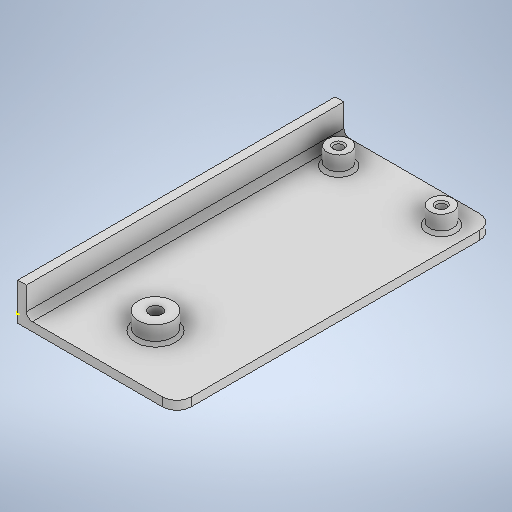
# Autodesk Inventor part: long_protoboard_backplate
Saved by Autodesk Inventor 2025.2 (Build 292293000, 293)
## iProperties
Created: 2025-03-28
Part Number: long_protoboard_backplate
Material: Generic
Document SubType Name: Modeling
Designer: osmon
Density: 1 g/cm^3
Appearance: Default
Author: osmon
Autodesk Inventor part; units mm, degrees
ref_plane "YZ Plane" through (0, 0, 0) normal (1, 0, 0) x (0, 1, 0)
ref_plane "XZ Plane" through (0, 0, 0) normal (0, 1, 0) x (-1, 0, 0)
ref_plane "XY Plane" through (0, 0, 0) normal (0, 0, 1) x (1, 0, 0)
sketch "Sketch1" plane through (0, 0, 0) normal (0, 1, 0) x (-1, 0, 0)
  line L0 (0, 0) -> (-55.1, 0)
  line L1 (-55.1, 0) -> (-55.1, -110)
  line L2 (-55.1, -110) -> (0, -110)
  line L3 (0, -110) -> (0, 0)
  dimension "d0" = 110
  dimension "d28" = 55.1
  constraints: 8 end point, 2 parallel, 1 horizontal, 1 perpendicular
  measures "d0" distance of L1.end L0.end
  measures "d28" distance of L1.end L2.end
extrude "Extrusion1" add sketch "Sketch1" along normal blind 3
sketch "Sketch2" plane through (0, 3, 0) normal (0, 1, 0) x (1, 0, 0)
  line L0 (55.1, 0) -> (55.1, 110) projected
  line L1 (55.1, 110) -> (0, 110) projected
  line L2 (0, 110) -> (0, 0) projected
  line L3 (0, 0) -> (55.1, 0) projected
  circle A0 centre (11.25, 99.95) radius 4
  circle A1 centre (46.85, 99.95) radius 4
  circle A2 centre (29.05, 18.6623) radius 6
  point P0 (27.55, 110)
  dimension "d3" = 8
  dimension "d4" = 10.05
  dimension "d6" = 8
  dimension "d7" = 10.05
  dimension "d8" = 8.25
  dimension "d29" = 12
  dimension "d30" = 91.35
  dimension "d39" = 26.05
  dimension "d40" = 35.6
  constraints: 3 centre point, 1 midpoint
  measures "d3" diameter of A0
  measures "d4" distance from line of L1 A0.centre
  measures "d6" diameter of A1
  measures "d7" distance from line of L1 A1.centre
  measures "d8" distance from line of L0 A1.centre
  measures "d29" diameter of A2
  measures "d30" distance of point (27.55, 110) A2.centre
  measures "d39" distance from line of L0 A2.centre
  measures "d40" distance of A1.centre A0.centre
extrude "Extrusion2" cut sketch "Sketch2" against normal blind 0.5 contours A0 | A1 | A2
sketch "Sketch3" plane through (11.25, 2.5, -99.95) normal (0, 1, 0) x (1, 0, 0)
  circle A0 centre (0, 0) radius 4 projected
  circle A1 centre (0, 0) radius 4
  circle A2 centre (35.6, 0) radius 4 projected
  circle A3 centre (35.6, 0) radius 4
  circle A4 centre (17.8, -81.2877) radius 6 projected
  circle A5 centre (17.8, -81.2877) radius 6
  point P0 (-11.25, -99.95)
  dimension "d32" = 12
  constraints: 3 centre point, 3 coincident, 2 concentric
  measures "d32" diameter of A5
extrude "Extrusion3" add sketch "Sketch3" along normal blind 6.5
sketch "Sketch4" plane through (11.25, 9, -99.95) normal (0, 1, 0) x (1, 0, 0)
  circle A0 centre (0, 0) radius 4 projected
  circle A1 centre (0, 0) radius 1.5
  circle A2 centre (35.6, 0) radius 4 projected
  circle A3 centre (35.6, 0) radius 1.5
  point P0 (-11.25, -99.95)
  dimension "d13" = 3
  dimension "d14" = 3
  constraints: 2 centre point, 2 coincident
  measures "d13" diameter of A1
  measures "d14" diameter of A3
extrude "Extrusion4" cut sketch "Sketch4" against normal blind 3.7 contours A1 | A3
chamfer "Chamfer1" distance 1 angle 45 3 edges at (7.25, 3, -99.95) (42.85, 3, -99.95) (23.05, 3, -18.6623)
chamfer "Chamfer2" distance 0.5 angle 45 2 edges at (9.75, 9, -99.95) (45.35, 9, -99.95)
sketch "Sketch5" plane through (0, 3, 0) normal (0, 1, 0) x (1, 0, 0)
  circle A0 centre (11.25, 99.95) radius 1.5 projected
  point P0 (0, 0)
sketch "Sketch6" plane through (11.25, 5.3, -99.95) normal (0, 1, 0) x (1, 0, 0)
  circle A0 centre (0, 0) radius 1.5 projected
  circle A1 centre (0, 0) radius 1.1
  circle A2 centre (35.6, 0) radius 1.5 projected
  circle A3 centre (35.6, 0) radius 1.1
  point P0 (-11.25, -99.95)
  dimension "d23" = 2.2
  dimension "d24" = 2.2
  constraints: 2 centre point, 2 coincident
  measures "d23" diameter of A1
  measures "d24" diameter of A3
extrude "Extrusion5" cut sketch "Sketch6" against normal blind 1.3 contours A1 | A3
sketch "Sketch7" plane through (29.05, 9, -18.6623) normal (0, 1, 0) x (1, 0, 0)
  circle A0 centre (0, 0) radius 2.25
  point P0 (-29.05, -18.6623)
  dimension "d33" = 4.5
  constraints: 1 centre point
  measures "d33" diameter of A0
extrude "Extrusion6" cut sketch "Sketch7" against normal blind 4.2
sketch "Sketch8" plane through (29.05, 4.8, -18.6623) normal (0, 1, 0) x (1, 0, 0)
  circle A0 centre (0, 0) radius 2.25 projected
  circle A1 centre (0, 0) radius 1.6
  point P0 (-29.05, -18.6623)
  dimension "d36" = 3.2
  constraints: 1 centre point, 1 coincident
  measures "d36" diameter of A1
extrude "Extrusion7" cut sketch "Sketch8" against normal blind 1.8 contours A1
sketch "Sketch9" plane through (0, 3, 0) normal (0, 1, 0) x (1, 0, 0)
  circle A0 centre (46.85, 99.95) radius 5 projected
  line L0 (55.1, 0) -> (55.1, 110) projected
  line L1 (55.1, 110) -> (0, 110) projected
  line L2 (0, 110) -> (0, 0) projected
  line L3 (0, 0) -> (55.1, 0) projected
  circle A1 centre (11.25, 99.95) radius 5 projected
  circle A2 centre (29.05, 18.6623) radius 7 projected
  line L4 (55.1, 110) -> (0, 110) projected
  line L5 (0, 110) -> (3, 110)
  line L6 (3, 110) -> (3, 0)
  line L7 (3, 0) -> (0, 0)
  line L8 (0, 0) -> (0, 110)
  dimension "d41" = 3
  constraints: 8 end point, 2 parallel, 1 horizontal, 1 perpendicular, 1 point on line
  measures "d41" distance of L6.end L7.end
extrude "Extrusion8" add sketch "Sketch9" along normal blind 10 contours L3 L2 L1 L6
fillet "Fillet2" radius 5 2 edges at (55.1, 1.5, -110) (55.1, 1.5, 0)
fillet "Fillet3" radius 2 1 edges at (3, 3, -55)
body "Solid1"
